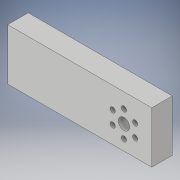
# Autodesk Inventor part: core hex motor to 30x30 mount
Saved by Autodesk Inventor 2019 (Build 230136000, 136)
## iProperties
Created: 2017-12-08
Part Number: core hex motor to 30x30 mount
Material: Generic
Document SubType Name: Modeling
Designer: User
Density: 1 g/cm^3
Appearance: Default
Author: User
Autodesk Inventor part; units mm, degrees
ref_plane "YZ Plane" through (0, 0, 0) normal (1, 0, 0) x (0, 1, 0)
ref_plane "XZ Plane" through (0, 0, 0) normal (0, 1, 0) x (-1, 0, 0)
ref_plane "XY Plane" through (0, 0, 0) normal (0, 0, 1) x (1, 0, 0)
sketch "Sketch1" plane through (0, 0, 0) normal (0, 0, 1) x (1, 0, 0)
  line L0 (0, 0) -> (63.5, 0)
  line L1 (63.5, 0) -> (63.5, 31.75)
  line L2 (63.5, 31.75) -> (0, 31.75)
  line L3 (0, 31.75) -> (0, 0)
  dimension "d0" = 63.5
  dimension "d1" = 31.75
  constraints: 8 end point, 2 parallel, 1 horizontal, 1 perpendicular
  measures "d0" distance of L2.end L1.end
  measures "d1" distance of L1.end L0.end
extrude "Extrusion1" add sketch "Sketch1" along normal blind 12.7
sketch "Sketch2" plane through (0, 0, 12.7) normal (0, 0, 1) x (1, 0, 0)
  line L0 (63.5, 0) -> (63.5, 31.75) projected
  line L1 (63.5, 12.7901) -> (80.6196, 12.7901) construction
  line L2 (0, 0) -> (63.5, 0) projected
  line L3 (46.3804, 0) -> (46.3804, 14.605)
  line L4 (46.3804, 0) -> (60.9854, 0) construction
  circle A0 centre (46.3804, 14.605) radius 3.4925
  circle A1 centre (46.3804, 14.605) radius 8.001
  circle A2 centre (46.3804, 6.604) radius 1.5875
  circle A3 centre (53.3095, 10.6045) radius 1.5875
  circle A4 centre (46.3804, 14.605) radius 8.001
  circle A5 centre (53.3095, 18.6055) radius 1.5875
  circle A6 centre (46.3804, 14.605) radius 8.001
  circle A7 centre (46.3804, 22.606) radius 1.5875
  circle A8 centre (46.3804, 14.605) radius 8.001
  circle A9 centre (39.4513, 18.6055) radius 1.5875
  circle A10 centre (46.3804, 14.605) radius 8.001
  circle A11 centre (39.4513, 10.6045) radius 1.5875
  circle A12 centre (46.3804, 14.605) radius 8.001
  dimension "d9" = 16.002
  dimension "d6" = 14.605
  dimension "d7" = 90
  dimension "d8" = 6.985
  dimension "d10" = 3.175
  dimension "d13" = 360
  dimension "d17" = 17.1196
  constraints: 7 centre point, 6 end point, 3 point on line, 2 coincident, 2 horizontal, 2 perpendicular, 2 vertical alignment, 41 other
  measures "d6" distance of L3.start L3.end
  measures "d7" angle of L4 L3
  measures "d8" diameter of A0
  measures "d10" diameter of A2
  measures "d17" distance from line of L0 L3.end
extrude "Extrusion2" cut sketch "Sketch2" against normal blind 19.05 contours A2 A1 L3 | L3 A1 A2 | A1 A2 L3 | L3 A2 A1 | A11 A1 | A1 A11 | A3 A1 | A1 A3 | A9 A1 | A1 A9 | A5 A1 | A1 A5 | A7 A1 | A1 A7 | A0
thicken "Thicken1" operation add thickness 25.4 both sides no extend neighbours yes toward (-1, 0, 0) faces at (0, 21.1667, 4.2333)
sketch "Sketch4" plane through (63.5, 0, 0) normal (0, -1, 0) x (1, 0, 0)
  line L0 (-88.9, 0) -> (-88.9, 12.7) projected
  line L1 (0, 0) -> (0, 12.7) projected
  point P0 (-63.5, 0)
  point P1 (-82.55, 6.35)
  point P2 (-44.45, 6.35)
  point P3 (-6.35, 6.35)
  dimension "d42" = 6.35
  dimension "d43" = 88.9
  dimension "d44" = 44.45
  dimension "d45" = 6.35
  measures "d42" distance from line of L0 point (-82.55, 6.35)
  measures "d43" distance from line of L1 L0.end
  measures "d44" distance from line of L1 point (-44.45, 6.35)
  measures "d45" distance from line of L1 point (-6.35, 6.35)
hole "Hole1" at (-19.05, 0, 6.35) at (19.05, 0, 6.35) at (57.15, 0, 6.35) direction (0, 1, 0) diameter 3.302 depth 7.62 tip angle 118 thread size "8-32 UNC" class "2B" standard "ANSI Unified Screw Threads"
equation "\"d44\" = 0.5 * d43"
body "Solid1"
